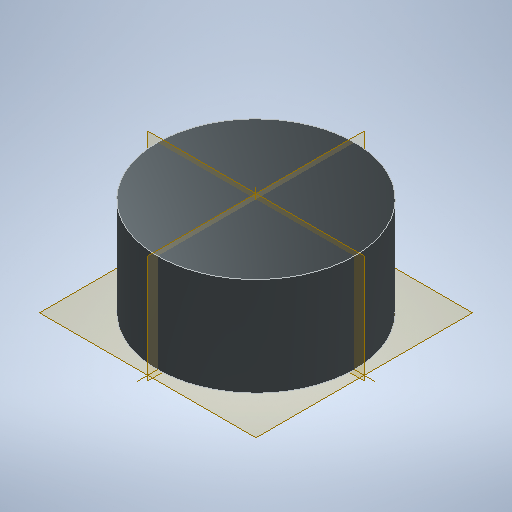
# Autodesk Inventor part: magnet10_5
Saved by Autodesk Inventor 2025.2 (Build 292293000, 293)
## iProperties
Created: 2025-03-15
Part Number: magnet10_5
Material: Iron, Ductile
Document SubType Name: Modeling
Designer: yehorderehus
Density: 7.15 g/cm^3
Appearance: Iron Gray
Author: yehorderehus
Autodesk Inventor part; units mm, degrees
sketch "Sketch1" plane through (0, 0, 0) normal (0, 1, 0) x (-1, 0, 0)
  circle A0 centre (0, 0) radius 5
  dimension "d0" = 10
  constraints: 1 centre point, 1 coincident
  measures "d0" diameter of A0
extrude "Extrusion1" add sketch "Sketch1" along normal blind 5
body "Solid1"
